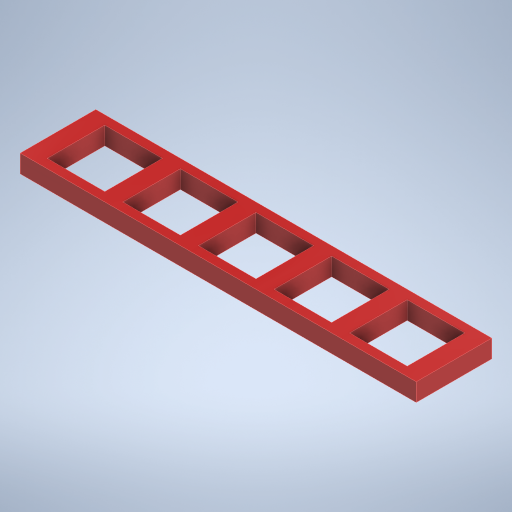
# Autodesk Inventor part: Slide
Saved by Autodesk Inventor 2024 (Build 280153000, 153)
## iProperties
Created: 2023-10-03
Part Number: Slide
Material: Generic
Document SubType Name: Modeling
Designer: flynf
Density: 1 g/cm^3
Appearance: Red
Author: flynf
Autodesk Inventor part; units mm, degrees
ref_plane "YZ Plane" through (0, 0, 0) normal (1, 0, 0) x (0, 1, 0)
ref_plane "XZ Plane" through (0, 0, 0) normal (0, 1, 0) x (-1, 0, 0)
ref_plane "XY Plane" through (0, 0, 0) normal (0, 0, 1) x (1, 0, 0)
sketch "Sketch1" plane through (0, 0, 0) normal (0, 1, 0) x (-1, 0, 0)
  line L0 (0, 0) -> (279.4, 0)
  line L1 (279.4, 0) -> (279.4, 53.34)
  line L2 (279.4, 53.34) -> (0, 53.34)
  line L3 (0, 53.34) -> (0, 0)
  constraints: 8 end point, 2 parallel, 1 horizontal, 1 perpendicular
extrude "Extrusion1" add sketch "Sketch1" along normal blind 12.7
sketch "Sketch2" plane through (0, 12.7, 0) normal (0, 1, 0) x (1, 0, 0)
  line L0 (-12.7, -46.99) -> (-53.34, -46.99)
  line L1 (-53.34, -46.99) -> (-53.34, -6.35)
  line L2 (-53.34, -6.35) -> (-12.7, -6.35)
  line L3 (-12.7, -6.35) -> (-12.7, -46.99)
  line L4 (-279.4, -53.34) -> (0, -53.34) projected
  line L5 (0, -53.34) -> (0, 0) projected
  line L6 (-66.04, -46.99) -> (-106.68, -46.99)
  line L7 (-106.68, -46.99) -> (-106.68, -6.35)
  line L8 (-106.68, -6.35) -> (-66.04, -6.35)
  line L9 (-66.04, -6.35) -> (-66.04, -46.99)
  line L10 (-119.38, -46.99) -> (-160.02, -46.99)
  line L11 (-160.02, -46.99) -> (-160.02, -6.35)
  line L12 (-160.02, -6.35) -> (-119.38, -6.35)
  line L13 (-119.38, -6.35) -> (-119.38, -46.99)
  line L14 (-172.72, -46.99) -> (-213.36, -46.99)
  line L15 (-213.36, -46.99) -> (-213.36, -6.35)
  line L16 (-213.36, -6.35) -> (-172.72, -6.35)
  line L17 (-172.72, -6.35) -> (-172.72, -46.99)
  line L18 (-226.06, -46.99) -> (-266.7, -46.99)
  line L19 (-266.7, -46.99) -> (-266.7, -6.35)
  line L20 (-266.7, -6.35) -> (-226.06, -6.35)
  line L21 (-226.06, -6.35) -> (-226.06, -46.99)
  dimension "d2" = 40.64
  dimension "d3" = 40.64
  dimension "d4" = 6.35
  dimension "d5" = 12.7
  dimension "d6" = 40.64
  dimension "d7" = 12.7
  dimension "d8" = 40.64
  dimension "d9" = 12.7
  dimension "d10" = 40.64
  dimension "d11" = 12.7
  dimension "d12" = 40.64
  dimension "d13" = 12.7
  constraints: 40 end point, 10 parallel, 5 horizontal, 5 perpendicular
  measures "d2" distance of L1.end L2.end
  measures "d3" distance of L0.end L1.end
  measures "d4" distance between parallel lines of L4 L0
  measures "d5" distance between parallel lines of L3 L5
  measures "d6" distance of L7.end L8.end
  measures "d7" distance between parallel lines of L9 L1
  measures "d8" distance of L11.end L12.end
  measures "d9" distance between parallel lines of L13 L7
  measures "d10" distance of L15.end L16.end
  measures "d11" distance between parallel lines of L17 L11
  measures "d12" distance of L19.end L20.end
  measures "d13" distance between parallel lines of L21 L15
extrude "Extrusion2" cut sketch "Sketch2" against normal through all
body "Solid1"
